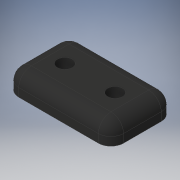
# Autodesk Inventor part: Heated Bed Belt Clamp
Saved by Autodesk Inventor 2019.4 (Build 234330000, 330)
## iProperties
Created: 2019-05-18
Part Number: Heated Bed Belt Clamp
Material: ABS Plastic
Document SubType Name: Modeling
Designer: Richard Hall
Density: 1.06 g/cm^3
Appearance: Rubber - Black
Author: Richard Hall
Autodesk Inventor part; units mm, degrees
ref_plane "YZ Plane" through (0, 0, 0) normal (1, 0, 0) x (0, 1, 0)
ref_plane "XZ Plane" through (0, 0, 0) normal (0, 1, 0) x (-1, 0, 0)
ref_plane "XY Plane" through (0, 0, 0) normal (0, 0, 1) x (1, 0, 0)
sketch "Sketch1" plane through (0, 0, 0) normal (0, 1, 0) x (-1, 0, 0)
  line L0 (9.5, 7.5) -> (-9.5, 7.5)
  line L1 (-12.5, 4.5) -> (-12.5, -4.5)
  line L2 (-9.5, -7.5) -> (9.5, -7.5)
  line L3 (12.5, -4.5) -> (12.5, 4.5)
  line L4 (12.5, 7.5) -> (-12.5, -7.5) construction
  line L5 (-12.5, 7.5) -> (12.5, -7.5) construction
  arc A0 (12.5, 4.5) -> (9.5, 7.5) centre (9.5, 4.5) ccw
  arc A1 (9.5, -7.5) -> (12.5, -4.5) centre (9.5, -4.5) ccw
  arc A2 (-12.5, -4.5) -> (-9.5, -7.5) centre (-9.5, -4.5) ccw
  arc A3 (-9.5, 7.5) -> (-12.5, 4.5) centre (-9.5, 4.5) ccw
  circle A4 centre (6, 0) radius 1.75
  circle A5 centre (-6, 0) radius 1.75
  point P0 (0, 0)
  point P1 (0, 0)
  dimension "d0" = 25
  dimension "d1" = 15
  dimension "d2" = 3
  dimension "d3" = 3.5
  dimension "d4" = 3.5
  dimension "d5" = 12
  dimension "d6" = 6
  constraints: 12 end point, 8 point on circle, 8 point on line, 8 tangent, 6 centre point, 3 equal radius, 3 midpoint, 2 horizontal alignment, 2 parallel, 1 horizontal, 1 perpendicular
  measures "d0" distance of L5.end L4.end
  measures "d1" distance of L4.end L5.start
  measures "d2" radius of A0
  measures "d3" diameter of A4
  measures "d4" diameter of A5
  measures "d5" distance of A5.centre A4.centre
  measures "d6" distance of point (0, 0) A4.centre
extrude "Extrusion1" add sketch "Sketch1" along normal mid plane 5
fillet "Fillet1" radius 3 8 edges at (11.6213, 2.5, 6.6213) (12.5, 2.5, 0) (11.6213, 2.5, -6.6213) (0, 2.5, -7.5) (-11.6213, 2.5, -6.6213) (-12.5, 2.5, 0) (-11.6213, 2.5, 6.6213) (0, 2.5, 7.5)
equation "\"d3\" = d4"
equation "\"d6\" = 0.5 * d5"
body "Solid1"
